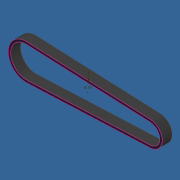
# Autodesk Inventor part: Bed_Unit_Belt
Saved by Autodesk Inventor 2020 (Build 240168000, 168)
## iProperties
Created: 2020-10-05
Part Number: Bed_Unit_Belt
Material: ゴム
Document SubType Name: Modeling
Designer: kenta iguchi
Density: 0.93 g/cm^3
Appearance: ゴム - 黒
Author: kenta iguchi
Autodesk Inventor part; units mm, degrees
ref_plane "YZ Plane" through (0, 0, 0) normal (1, 0, 0) x (0, 1, 0)
ref_plane "XZ Plane" through (0, 0, 0) normal (0, 1, 0) x (-1, 0, 0)
ref_plane "XY Plane" through (0, 0, 0) normal (0, 0, 1) x (1, 0, 0)
sketch "スケッチ1" plane through (0, 0, 0) normal (0, 0, 1) x (1, 0, 0)
  arc A0 (0.4093, 9.291) -> (0.4092, -9.291) centre (0, 0) ccw
  arc A1 (0.4752, 10.7895) -> (0.4752, -10.7895) centre (0, 0) ccw
  arc A2 (75.33, -7.4927) -> (75.33, 7.4927) centre (75, 0) ccw
  line L0 (0.4752, 10.7895) -> (75.33, 7.4927)
  line L1 (75.33, -7.4927) -> (0.4752, -10.7895)
  line L2 (75.1922, 5.9969) -> (0.4093, 9.291)
  circle A3 centre (75, 0) radius 6
  line L3 (0.4092, -9.291) -> (75.264, -5.9942)
  point P0 (1.0111, -13.9634)
  point P1 (90.5417, -7.4804)
  point P2 (90.5417, 7.4804)
  point P3 (1.0111, 13.9634)
  point P4 (0.9028, 12.4674)
  dimension "d0" = 18.6
  dimension "d2" = 75
  dimension "d3" = 1.5
  dimension "d7" = 12
  dimension "d8" = 1.5
  constraints: 8 end point, 8 point on circle, 7 tangent, 4 centre point, 2 coincident, 1 horizontal alignment
  measures "d0" diameter of A0
  measures "d2" distance of point (0, 0) A2.centre
  measures "d3" radial gap between concentric circles of A0 A1
  measures "d7" diameter of A3
  measures "d8" radial gap between concentric circles of A2 A3
extrude "押し出し1" add sketch "スケッチ1" along normal blind 6
sketch "スケッチ3" plane through (0, 0, 6) normal (0, 0, 1) x (1, 0, 0)
  arc A0 (75.33, -7.4927) -> (75.33, 7.4927) centre (75, 0) ccw projected
  line L0 (75.33, 7.4927) -> (0.4752, 10.7895) projected
  arc A1 (0.4752, 10.7895) -> (0.4752, -10.7895) centre (0, 0) ccw projected
  line L1 (0.4752, -10.7895) -> (75.33, -7.4927) projected
  arc A2 (0.4093, 9.291) -> (0.4092, -9.291) centre (0, 0) ccw projected
  line L2 (0.4093, 9.291) -> (75.1922, 5.9969) projected
  arc A3 (75.264, -5.9942) -> (75.1922, 5.9969) centre (75, 0) ccw projected
  line L3 (75.264, -5.9942) -> (0.4092, -9.291) projected
  line L4 (75.2208, 6.7464) -> (0.4423, 10.0403)
  arc A4 (0.4423, 10.0403) -> (0.4422, -10.0403) centre (0, 0) ccw
  line L5 (0.4422, -10.0403) -> (75.297, -6.7435)
  arc A5 (75.297, -6.7435) -> (75.2208, 6.7464) centre (75, 0) ccw
  dimension "d10" = 0.75
  constraints: 4 end point, 4 point on circle, 2 centre point, 3 other
  measures "d10" distance between parallel lines of L2 L4
